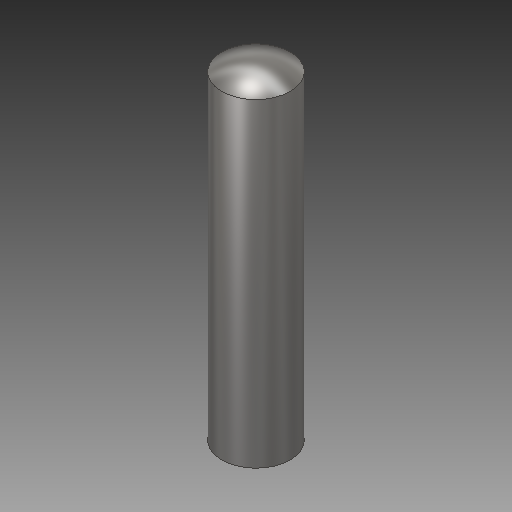
# Autodesk Inventor part: P1207.030-014
Saved by Autodesk Inventor 2019 (Build 230136000, 136)
## iProperties
Created: 2018-04-23
Part Number: P1207.030-014
Material: Stainless Steel AISI 317
Document SubType Name: Modeling
Designer: IEUser
Density: 8 g/cm^3
Appearance: Semi-Polished
Mass: 0.817892 g
Surface Area: 1.47356 cm^2
Volume: 0.102236 cm^3
Author: IEUser
Autodesk Inventor part; units mm, degrees
ref_plane "YZ Plane" through (0, 0, 0) normal (1, 0, 0) x (0, 1, 0)
ref_plane "XZ Plane" through (0, 0, 0) normal (0, 1, 0) x (-1, 0, 0)
ref_plane "XY Plane" through (0, 0, 0) normal (0, 0, 1) x (1, 0, 0)
sketch "Body Revolution Profile" plane through (0, 0, 0) normal (0, 0, 1) x (1, 0, 0)
  line L0 (0, 7.45) -> (0, -7.45)
  line L1 (1.5, 7) -> (1.5, -7)
  arc A0 (1.5, 7) -> (0, 7.45) centre (0, 4.725) ccw
  arc A1 (0, -7.45) -> (1.5, -7) centre (0, -4.725) ccw
  point P0 (0, 0)
  dimension "d0" = 14
  dimension "d1" = 0.45
  dimension "d2" = 0.45
  dimension "d3" = 7
  dimension "d4" = 0
  dimension "d5" = 1.5
  constraints: 4 end point, 4 point on circle, 2 centre point, 2 line through centre, 1 parallel, 1 vertical
  measures "d0" distance of L1.start L1.end
  measures "d1" vertical distance of L1.start L0.start
  measures "d2" vertical distance of L1.end L0.end
  measures "d3" vertical distance of point (0, 0) L1.start
  measures "d4" distance from line of point (0, 0) L0
  measures "d5" distance between parallel lines of L1 L0
revolve "Body" add sketch "Body Revolution Profile" angle 360 about axis through (0, 7.45, 0) along (0, -1, 0)
equation "\"d2\" = d1"
equation "\"d3\" = 0.5 * d0"
body "Solid1"
